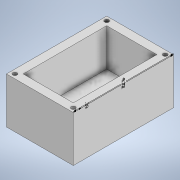
# Autodesk Inventor part: Water_Proof_Box_Bottom
Saved by Autodesk Inventor 2022 (Build 260153000, 153)
## iProperties
Created: 2023-07-12
Part Number: Water_Proof_Box_Bottom
Material: Generic
Document SubType Name: Modeling
Designer: jtw4137
Density: 1 g/cm^3
Appearance: Default
Author: jtw4137
Autodesk Inventor part; units mm, degrees
ref_plane "YZ Plane" through (0, 0, 0) normal (1, 0, 0) x (0, 1, 0)
ref_plane "XZ Plane" through (0, 0, 0) normal (0, 1, 0) x (-1, 0, 0)
ref_plane "XY Plane" through (0, 0, 0) normal (0, 0, 1) x (1, 0, 0)
sketch "Sketch1" plane through (0, 0, 0) normal (0, 1, 0) x (-1, 0, 0)
  line L0 (59.2038, 31.922) -> (59.2038, -88.078)
  line L1 (59.2038, -88.078) -> (-20.7962, -88.078)
  line L2 (-20.7962, -88.078) -> (-20.7962, 31.922)
  line L3 (-20.7962, 31.922) -> (59.2038, 31.922)
  point P0 (0, 0)
  dimension "d0" = 120
  dimension "d1" = 80
  constraints: 8 end point, 2 perpendicular, 1 vertical
  measures "d0" distance of L0.start L0.end
  measures "d1" distance of L2.end L0.start
extrude "Extrusion1" add sketch "Sketch1" along normal blind 55
shell "Shell2" thickness 10 removed faces 1 at (-5.8705, 55, -48.078)
sketch "Sketch12" plane through (0, 55, 0) normal (0, 1, 0) x (1, 0, 0)
  line L0 (10.7962, 78.078) -> (10.7962, -21.922) projected
  line L1 (10.7962, -21.922) -> (20.7962, -21.922)
  line L2 (20.7962, -31.922) -> (20.7962, 88.078) projected
  line L3 (20.7962, -21.922) -> (20.7962, -31.922)
  line L4 (20.7962, -31.922) -> (10.7962, -31.922)
  line L5 (10.7962, -31.922) -> (10.7962, -21.922)
  line L6 (20.7962, -31.922) -> (15.8432, -31.922)
  line L7 (-59.2038, -31.922) -> (20.7962, -31.922) projected
  line L8 (15.8432, -26.969) -> (20.7962, -26.969)
  line L9 (15.8432, -26.969) -> (15.8432, -31.922)
  point P0 (0, 0)
  dimension "d124" = 4.953
  dimension "d125" = 4.953
  constraints: 14 end point, 5 perpendicular, 2 point on line, 1 horizontal
  measures "d124" distance of L8.start L6.end
  measures "d125" distance of L8.start L8.end
hole "Hole11" at (15.8432, 55, 26.969) direction (0, -1, 0) diameter 5 end through all
sketch "Sketch19" plane through (0, 55, 0) normal (0, 1, 0) x (1, 0, 0)
  line L0 (10.7962, -21.922) -> (-49.2038, -21.922) projected
  line L1 (-49.2038, -21.922) -> (-49.2038, -31.922)
  line L2 (-59.2038, -31.922) -> (20.7962, -31.922) projected
  line L3 (-59.2038, -31.922) -> (-59.2038, -21.922)
  line L4 (-59.2038, 88.078) -> (-59.2038, -31.922) projected
  line L5 (-49.2038, -23.8125) -> (-49.2038, -21.922)
  line L6 (-59.2038, -21.922) -> (-49.2038, -21.922)
  line L7 (-49.2038, -21.922) -> (-49.2038, 78.078) projected
  line L8 (-49.2038, -21.922) -> (-54.2038, -21.922)
  line L9 (-54.1566, -26.875) -> (-49.2038, -26.922)
  line L10 (-54.1566, -26.875) -> (-54.2038, -21.922)
  point P0 (0, 0)
  dimension "d133" = 4.953
  dimension "d134" = 4.953
  constraints: 14 end point, 3 point on line, 2 midpoint, 1 parallel, 1 perpendicular, 1 vertical
  measures "d133" distance of L9.start L9.end
  measures "d134" vertical distance of L9.start L8.end
hole "Hole12" at (-54.1566, 55, 26.875) direction (0, -1, 0) diameter 5 end through all
sketch "Sketch21" plane through (0, 55, 0) normal (0, 1, 0) x (1, 0, 0)
  line L0 (10.7962, -21.922) -> (10.7962, 78.078) projected
  line L1 (10.7962, 78.078) -> (20.7962, 78.078)
  line L2 (20.7962, -31.922) -> (20.7962, 88.078) projected
  line L3 (20.7962, 88.078) -> (10.7962, 88.078)
  line L4 (20.7962, 88.078) -> (-59.2038, 88.078) projected
  line L5 (10.7962, 78.078) -> (10.7962, 88.078)
  line L6 (10.7962, 78.078) -> (-49.2038, 78.078) projected
  line L7 (10.7962, 78.078) -> (15.7962, 78.078)
  line L8 (15.8432, 83.031) -> (20.7962, 83.031)
  line L9 (15.8432, 83.031) -> (15.7962, 78.078)
  point P0 (0, 0)
  dimension "d146" = 4.953
  constraints: 12 end point, 3 point on line, 2 perpendicular, 1 horizontal, 1 midpoint
  measures "d146" distance of L8.start L8.end
hole "Hole13" at (15.8432, 55, -83.031) direction (0, -1, 0) diameter 5 end through all
sketch "Sketch22" plane through (0, 55, 0) normal (0, 1, 0) x (1, 0, 0)
  line L0 (-49.2038, 78.078) -> (10.7962, 78.078) projected
  line L1 (-49.2038, 78.078) -> (-59.2038, 78.078)
  line L2 (-59.2038, 88.078) -> (-59.2038, -31.922) projected
  line L3 (-59.2038, 88.078) -> (-49.2038, 88.078)
  line L4 (20.7962, 88.078) -> (-59.2038, 88.078) projected
  line L5 (-49.2038, 78.078) -> (-49.2038, 88.078)
  line L6 (-49.2038, 78.078) -> (-54.2038, 78.078)
  line L7 (-54.1568, 83.031) -> (-49.2038, 83.031)
  line L8 (-54.1568, 83.031) -> (-54.2038, 78.078)
  point P0 (0, 0)
  dimension "d155" = 4.953
  dimension "d156" = 4.953
  constraints: 12 end point, 3 point on line, 2 perpendicular, 1 horizontal, 1 midpoint
  measures "d155" distance of L7.start L7.end
  measures "d156" vertical distance of L7.start L6.end
hole "Hole14" at (-54.1568, 55, -83.031) direction (0, -1, 0) diameter 5 end through all
body "Solid1"
